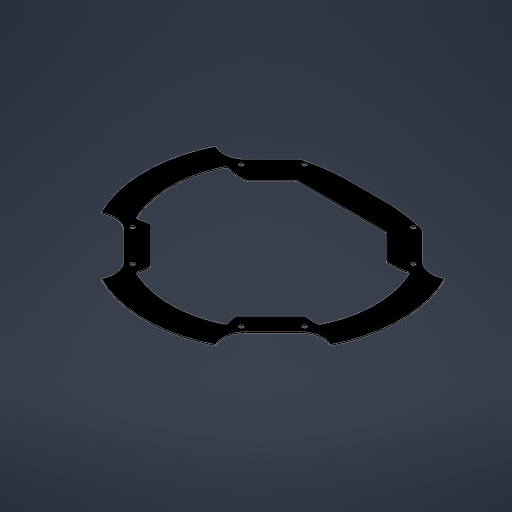
# Autodesk Inventor part: MettalringUnten_v3
Saved by Autodesk Inventor 2023.2 (Build 272271030, 271C)
## iProperties
Created: 2022-10-10
Part Number: MettalringUnten_v3
Material: Generic
Document SubType Name: Modeling
Designer: braun
Density: 1 g/cm^3
Appearance: Default
Author: braun
Autodesk Inventor part; units mm, degrees
ref_plane "YZ Plane" through (0, 0, 0) normal (1, 0, 0) x (0, 1, 0)
ref_plane "XZ Plane" through (0, 0, 0) normal (0, 1, 0) x (-1, 0, 0)
ref_plane "XY Plane" through (0, 0, 0) normal (0, 0, 1) x (1, 0, 0)
sketch "Sketch1" plane through (0, 0, 0) normal (0, 1, 0) x (-1, 0, 0)
  arc A0 (43.0581, -98.5) -> (-43.0581, -98.5) centre (0, 0) ccw
  line L0 (0, -107.5) -> (0, -98.5) construction
  line L1 (-18.0581, -73.5) -> (18.0581, -73.5)
  arc A1 (-18.0581, -73.5) -> (-43.0581, -98.5) centre (-18.0581, -98.5) ccw
  line L2 (0, 107.5) -> (0, 97.5) construction
  line L3 (0, 97.5) -> (-22.5, 97.5) construction
  line L4 (-22.5, 97.5) -> (-22.5, 82.5) construction
  line L5 (22.5, 90) -> (-22.5, 90) construction
  line L6 (15, 97.5) -> (-15, 97.5)
  line L7 (-15, 82.5) -> (15, 82.5)
  arc A2 (15, 82.5) -> (15, 97.5) centre (15, 90) ccw
  arc A3 (-15, 97.5) -> (-15, 82.5) centre (-15, 90) ccw
  line L8 (17.5, 82.5) -> (17.5, 77.5) construction
  circle A4 centre (17.5, 77.5) radius 1.6
  circle A5 centre (-17.5, 77.5) radius 1.6
  line L9 (-58.3363, 79.5495) -> (-79.5495, 58.3363)
  arc A6 (-47.7297, 68.9429) -> (-58.3363, 79.5495) centre (-53.033, 74.2462) ccw
  arc A7 (-79.5495, 58.3363) -> (-68.9429, 47.7297) centre (-74.2462, 53.033) ccw
  line L10 (-68.9429, 47.7297) -> (-47.7297, 68.9429)
  circle A8 centre (-67.1751, 42.4264) radius 1.6
  circle A9 centre (-42.4264, 67.1751) radius 1.6
  line L11 (-97.5, 15) -> (-97.5, -15)
  arc A10 (-82.5, 15) -> (-97.5, 15) centre (-90, 15) ccw
  arc A11 (-97.5, -15) -> (-82.5, -15) centre (-90, -15) ccw
  line L12 (-82.5, -15) -> (-82.5, 15)
  circle A12 centre (-77.5, -17.5) radius 1.6
  circle A13 centre (-77.5, 17.5) radius 1.6
  line L13 (-79.5495, -58.3363) -> (-58.3363, -79.5495)
  arc A14 (-68.9429, -47.7297) -> (-79.5495, -58.3363) centre (-74.2462, -53.033) ccw
  arc A15 (-58.3363, -79.5495) -> (-47.7297, -68.9429) centre (-53.033, -74.2462) ccw
  line L14 (-47.7297, -68.9429) -> (-68.9429, -47.7297)
  circle A16 centre (-42.4264, -67.1751) radius 1.6
  circle A17 centre (-67.1751, -42.4264) radius 1.6
  line L15 (-15, -97.5) -> (15, -97.5)
  arc A18 (-15, -82.5) -> (-15, -97.5) centre (-15, -90) ccw
  arc A19 (15, -97.5) -> (15, -82.5) centre (15, -90) ccw
  line L16 (15, -82.5) -> (-15, -82.5)
  circle A20 centre (17.5, -77.5) radius 1.6
  circle A21 centre (-17.5, -77.5) radius 1.6
  line L17 (58.3363, -79.5495) -> (79.5495, -58.3363)
  arc A22 (47.7297, -68.9429) -> (58.3363, -79.5495) centre (53.033, -74.2462) ccw
  arc A23 (79.5495, -58.3363) -> (68.9429, -47.7297) centre (74.2462, -53.033) ccw
  line L18 (68.9429, -47.7297) -> (47.7297, -68.9429)
  circle A24 centre (67.1751, -42.4264) radius 1.6
  circle A25 centre (42.4264, -67.1751) radius 1.6
  line L19 (97.5, -15) -> (97.5, 15)
  arc A26 (82.5, -15) -> (97.5, -15) centre (90, -15) ccw
  arc A27 (97.5, 15) -> (82.5, 15) centre (90, 15) ccw
  line L20 (82.5, 15) -> (82.5, -15)
  circle A28 centre (77.5, 17.5) radius 1.6
  circle A29 centre (77.5, -17.5) radius 1.6
  line L21 (79.5495, 58.3363) -> (58.3363, 79.5495)
  arc A30 (68.9429, 47.7297) -> (79.5495, 58.3363) centre (74.2462, 53.033) ccw
  arc A31 (58.3363, 79.5495) -> (47.7297, 68.9429) centre (53.033, 74.2462) ccw
  line L22 (47.7297, 68.9429) -> (68.9429, 47.7297)
  circle A32 centre (42.4264, 67.1751) radius 1.6
  circle A33 centre (67.1751, 42.4264) radius 1.6
  arc A34 (89.4718, -44.6631) -> (89.4718, 44.6631) centre (0, 0) ccw
  arc A35 (44.5267, 89.5398) -> (-44.6631, 89.4718) centre (0, 0) ccw
  line L23 (43.0581, -98.5) -> (48.0581, -98.5) construction
  circle A36 centre (48.0581, -88.5) radius 1.6
  circle A37 centre (-48.0581, -88.5) radius 1.6
  arc A38 (43.0581, -98.5) -> (18.0581, -73.5) centre (18.0581, -98.5) ccw
  arc A39 (-18.0581, -73.5) -> (-43.0581, -98.5) centre (-18.0581, -98.5) ccw
  circle A40 centre (0, 0) radius 103.75 construction
  circle A41 centre (30, 99.318) radius 1.6
  circle A42 centre (-30, 99.318) radius 1.6
  circle A43 centre (-99.318, 30) radius 1.6
  circle A44 centre (-99.318, -30) radius 1.6
  circle A45 centre (-30, -99.318) radius 1.6
  circle A46 centre (30, -99.318) radius 1.6
  circle A47 centre (99.318, -30) radius 1.6
  circle A48 centre (99.318, 30) radius 1.6
  line L24 (100, 0) -> (80, 0) construction
  arc A49 (71.6318, -35.6214) -> (71.6318, 35.6214) centre (0, 0) ccw
  line L25 (58.3363, -58.3363) -> (44.1942, -44.1942) construction
  line L26 (44.1942, -44.1942) -> (54.8008, -33.5876)
  line L27 (44.1942, 44.1942) -> (54.8008, 33.5876)
  line L28 (44.1942, 44.1942) -> (58.3363, 58.3363) construction
  line L29 (44.1942, 44.1942) -> (33.5876, 54.8008)
  arc A50 (-71.6318, 35.6214) -> (-71.6318, -35.6214) centre (0, 0) ccw
  line L30 (-44.1942, -44.1942) -> (-54.8008, -33.5876)
  line L31 (-44.1942, 44.1942) -> (-54.8008, 33.5876)
  arc A51 (-54.8008, 33.5876) -> (-71.6318, 35.6214) centre (-67.5275, -1.0734) ccw
  line L32 (-44.1942, 44.1942) -> (-33.5876, 54.8008)
  arc A52 (35.6214, 71.6318) -> (-35.6214, 71.6318) centre (0, 0) ccw
  line L33 (44.1942, -44.1942) -> (34.8883, -53.5)
  line L34 (-44.1942, -44.1942) -> (-34.8883, -53.5)
  line L35 (0, -73.5) -> (0, -53.5) construction
  line L36 (0, -53.5) -> (34.8883, -53.5)
  line L37 (0, -53.5) -> (-34.8883, -53.5)
  arc A53 (89.4718, -44.6631) -> (68.9429, -47.7297) centre (81.2792, -60.066) ccw
  arc A54 (68.9429, 47.7297) -> (89.4718, 44.6631) centre (81.2792, 60.066) ccw
  arc A55 (-68.9429, -47.7297) -> (-89.4718, -44.6631) centre (-81.2792, -60.066) ccw
  arc A56 (-89.4718, 44.6631) -> (-68.9429, 47.7297) centre (-81.2792, 60.066) ccw
  arc A57 (44.6631, 89.4718) -> (47.7297, 68.9429) centre (60.066, 81.2792) ccw
  arc A58 (-47.7297, 68.9429) -> (-44.6631, 89.4718) centre (-60.066, 81.2792) ccw
  arc A59 (18.0581, -73.5) -> (47.7297, -68.9429) centre (12.7356, 60.0312) ccw
  arc A60 (-47.7297, -68.9429) -> (-18.0581, -73.5) centre (-12.7356, 60.0312) ccw
  arc A61 (44.6631, 89.4718) -> (44.5267, 89.5398) centre (0, 0.0001) ccw
  arc A62 (35.6214, 71.6318) -> (33.5876, 54.8008) centre (70.2823, 58.9051) ccw
  arc A63 (54.8008, 33.5876) -> (71.6318, 35.6214) centre (58.9051, 70.2823) ccw
  arc A64 (71.6318, -35.6214) -> (54.8008, -33.5876) centre (58.9051, -70.2823) ccw
  arc A65 (-33.5876, 54.8008) -> (-35.6214, 71.6318) centre (-70.2823, 58.9051) ccw
  arc A66 (-54.8008, -33.5876) -> (-71.6318, -35.6214) centre (-58.9051, -70.2823) ccw
  arc A67 (-89.4718, 44.6631) -> (-89.4718, -44.6631) centre (0.0031, 0) ccw
  point P0 (0, 90)
  point P1 (-45.9619, 70.7107)
  point P2 (-82.5, 17.5)
  point P3 (-70.7107, -45.9619)
  point P4 (-17.5, -82.5)
  point P5 (45.9619, -70.7107)
  point P6 (82.5, -17.5)
  point P7 (70.7107, 45.9619)
  point P8 (35.7159, -76.7698)
  point P9 (-44.6631, 89.4718)
  dimension "d19" = 360
  dimension "d130" = 360
  dimension "d132" = 20
  dimension "d133" = 20
  dimension "d134" = 90
  dimension "d135" = 15
  dimension "d139" = 20
  constraints: 87 point on circle, 78 end point, 68 centre point, 26 symmetric about line, 11 point on line, 7 tangent, 5 midpoint, 4 vertical, 3 coincident, 3 horizontal, 1 parallel, 149 other
  measures "d132" distance of L24.start L24.end
  measures "d133" distance of L25.start L25.end
  measures "d134" angle of L18 L25
  measures "d135" distance of L25.end L26.end
  measures "d139" distance of L35.start L35.end
extrude "Extrusion8" add sketch "Sketch1" along normal blind 1 contours L1 A60 L14 A55 A67 A56 L10 A58 A35 A61 A57 L22 A54 A34 A53 L18 A59 | A2 L7 A3 L6 | A52 A4 | A52 A5 | A28 A49 | A29 A49 | A50 A13 | A50 A12 | A10 L12 A11 L11 | A26 L20 A27 L19 picked at (17.6978, 78.3761) picked at (-17.6978, 78.3761) picked at (78.3736, 17.7082) picked at (78.3736, -17.7082) picked at (-78.3761, 17.6978) picked at (-78.3761, -17.6978)
fillet "Fillet6" radius 2 18 edges at (-71.6318, 0.5, -35.6214) (-54.8008, 0.5, -33.5876) (-71.6318, 0.5, 35.6214) (-54.8008, 0.5, 33.5876) (-33.5876, 0.5, 54.8008) (-35.6214, 0.5, 71.6318) (35.6214, 0.5, 71.6318) (33.5876, 0.5, 54.8008) (54.8008, 0.5, 33.5876) (71.6318, 0.5, 35.6214) (71.6318, 0.5, -35.6214) (54.8008, 0.5, -33.5876) (34.8883, 0.5, -53.5) (-34.8883, 0.5, -53.5) (-47.7297, 0.5, -68.9429) (-18.0581, 0.5, -73.5) (18.0581, 0.5, -73.5) (47.7297, 0.5, -68.9429)
sketch "Sketch11" plane through (0, 1, 0) normal (0, 1, 0) x (1, 0, 0)
  line L0 (-34.0908, -54.2975) -> (-54.2975, -34.0908) projected
  line L1 (-44.1942, -44.1942) -> (-47.7297, -47.7297)
  line L2 (-68.9429, -47.7297) -> (-47.7297, -68.9429) projected
  line L3 (-47.7297, -47.7297) -> (-61.973, -33.4864)
  arc A0 (-55.5288, -33.5134) -> (-70.0005, -35.0652) centre (-58.9051, -70.2823) ccw projected
  line L4 (-47.7297, -47.7297) -> (-33.4864, -61.973)
  arc A1 (-35.0652, -70.0005) -> (-33.5134, -55.5288) centre (-70.2823, -58.9051) ccw projected
  arc A2 (-54.2975, -34.0908) -> (-55.5288, -33.5134) centre (-55.7117, -35.5051) ccw projected
  line L5 (-34.1542, -54.2341) -> (-54.2975, -34.0908)
  line L6 (0, -73.9408) -> (0, -70.0005)
  arc A3 (-33.5134, -55.5288) -> (-34.0908, -54.2975) centre (-35.5051, -55.7117) ccw projected
  arc A4 (-33.5134, -55.5288) -> (-34.0908, -54.2975) centre (-35.5051, -55.7117) ccw
  line L7 (34.0908, -54.2975) -> (54.2975, -34.0908)
  line L8 (44.1942, -44.1942) -> (47.7297, -47.7297)
  line L9 (47.7297, -47.7297) -> (61.973, -33.4864)
  line L10 (47.7297, -47.7297) -> (33.4864, -61.973)
  arc A5 (33.5134, -55.5288) -> (35.0652, -70.0005) centre (70.2823, -58.9051) ccw
  arc A6 (55.5288, -33.5134) -> (54.2975, -34.0908) centre (55.7117, -35.5051) ccw
  line L11 (34.1542, -54.2341) -> (54.2975, -34.0908)
  arc A7 (34.0908, -54.2975) -> (33.5134, -55.5288) centre (35.5051, -55.7117) ccw
  arc A8 (34.0908, -54.2975) -> (33.5134, -55.5288) centre (35.5051, -55.7117) ccw
  arc A9 (55.9547, -33.9897) -> (53.9136, -34.4747) centre (55.3278, -35.8889) ccw projected
  arc A10 (55.9547, -33.9897) -> (53.9136, -34.4747) centre (55.3278, -35.8889) ccw
  arc A11 (55.9547, -33.9897) -> (70.4863, -35.7315) centre (67.5275, 1.0734) ccw projected
  arc A12 (55.9547, -33.9897) -> (60.3196, -35.1398) centre (67.5275, 1.0734) ccw
  point P0 (0, 0)
  point P1 (47.7297, -68.9429)
  point P2 (58.9051, -70.2823)
  dimension "d145" = 5
  constraints: 20 end point, 18 point on circle, 16 symmetric about line, 7 centre point, 3 point on line, 2 perpendicular, 2 tangent, 1 midpoint, 1 parallel, 1 vertical, 4 other
  measures "d145" distance of L1.start L1.end
extrude "Extrusion9" cut sketch "Sketch11" against normal blind 1
fillet "Fillet7" radius 2 4 edges at (-33.4864, 0.5, 61.973) (-61.973, 0.5, 33.4864) (60.3196, 0.5, 35.1398) (33.4864, 0.5, 61.973)
body "Solid3"
